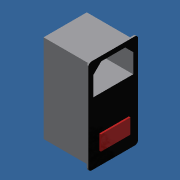
# Autodesk Inventor part: power
Saved by Autodesk Inventor 2018 (Build 220112000, 112)
## iProperties
Created: 2020-10-01
Part Number: power
Material: Generic
Document SubType Name: Modeling
Designer: Nathann
Density: 1 g/cm^3
Appearance: Default
Author: Nathann
Autodesk Inventor part; units mm, degrees
ref_plane "YZ Plane" through (0, 0, 0) normal (1, 0, 0) x (0, 1, 0)
ref_plane "XZ Plane" through (0, 0, 0) normal (0, 1, 0) x (-1, 0, 0)
ref_plane "XY Plane" through (0, 0, 0) normal (0, 0, 1) x (1, 0, 0)
sketch "Sketch1" plane through (0, 0, 0) normal (1, 0, 0) x (0, 1, 0)
  line L0 (0, 0) -> (27, 0)
  line L1 (27, 0) -> (27, -55)
  line L2 (27, -55) -> (0, -55)
  line L3 (0, -55) -> (0, 0)
  dimension "d0" = 27
  dimension "d1" = 55
  constraints: 8 end point, 2 parallel, 1 horizontal, 1 perpendicular
  measures "d0" distance of L0.start L0.end
  measures "d1" distance of L0.end L1.end
extrude "Extrusion1" add sketch "Sketch1" along normal blind 30
sketch "Sketch2" plane through (30, 0, 0) normal (1, 0, 0) x (0, 0, -1)
  line L0 (-2, 29) -> (57, 29)
  line L1 (57, 29) -> (57, -2)
  line L2 (57, -2) -> (-2, -2)
  line L3 (-2, -2) -> (-2, 29)
  line L4 (0, 27) -> (0, 0) projected
  line L5 (55, 27) -> (0, 27) projected
  line L6 (0, 0) -> (55, 0) projected
  line L7 (55, 0) -> (55, 27) projected
  dimension "d4" = 2
  dimension "d5" = 2
  dimension "d6" = 2
  dimension "d7" = 2
  constraints: 8 end point, 2 parallel, 1 horizontal, 1 perpendicular
  measures "d4" distance between parallel lines of L3 L4
  measures "d5" distance between parallel lines of L5 L0
  measures "d6" distance between parallel lines of L6 L2
  measures "d7" distance between parallel lines of L1 L7
extrude "Extrusion2" add sketch "Sketch2" against normal blind 1
fillet "Fillet1" radius 2 4 edges at (29.5, 29, 2) (29.5, 29, -57) (29.5, -2, -57) (29.5, -2, 2)
sketch "Sketch3" plane through (30, 0, 0) normal (1, 0, 0) x (0, 0, -1)
  line L0 (6, 1) -> (18, 1)
  line L1 (18, 1) -> (18, 26)
  line L2 (18, 26) -> (6, 26)
  line L3 (1, 26) -> (1, 1)
  line L4 (0, 29) -> (55, 29) projected
  line L5 (55, -2) -> (0, -2) projected
  line L6 (1, 21) -> (6, 26)
  line L7 (1, 6) -> (6, 1)
  line L8 (-2, 0) -> (-2, 27) projected
  point P0 (0, 0)
  dimension "d11" = 17
  dimension "d12" = 25
  dimension "d13" = 31
  dimension "d14" = 3
  dimension "d15" = 3
  dimension "d16" = 5
  dimension "d17" = 5
  dimension "d18" = 5
  dimension "d19" = 5
  constraints: 12 end point, 2 parallel, 2 perpendicular, 2 point on line, 1 horizontal
  measures "d11" distance of L1.end L3.start
  measures "d12" distance of L3.start L3.end
  measures "d13" distance between parallel lines of L4 L5
  measures "d14" distance between parallel lines of L0 L5
  measures "d15" distance between parallel lines of L8 L3
  measures "d16" horizontal distance of L2.end L6.start
  measures "d17" horizontal distance of L0.start L7.start
  measures "d18" horizontal distance of L0.start L7.start
  measures "d19" horizontal distance of L2.end L6.start
extrude "Extrusion3" cut sketch "Sketch3" against normal blind 20
sketch "Sketch4" plane through (30, 0, 0) normal (1, 0, 0) x (0, 0, -1)
  line L0 (48.7705, 23.2756) -> (39.4061, 23.2756)
  line L1 (39.4061, 23.2756) -> (39.4061, 4.8716)
  line L2 (39.4061, 4.8716) -> (48.7705, 4.8716)
  line L3 (48.7705, 4.8716) -> (48.7705, 23.2756)
  point P0 (0, 0)
  constraints: 8 end point, 2 parallel, 1 horizontal, 1 perpendicular
extrude "Extrusion4" add sketch "Sketch4" along normal blind 1
equation "\"d14\" = -0.5 * d12 + 0.5 * d13"
body "Solid1"
